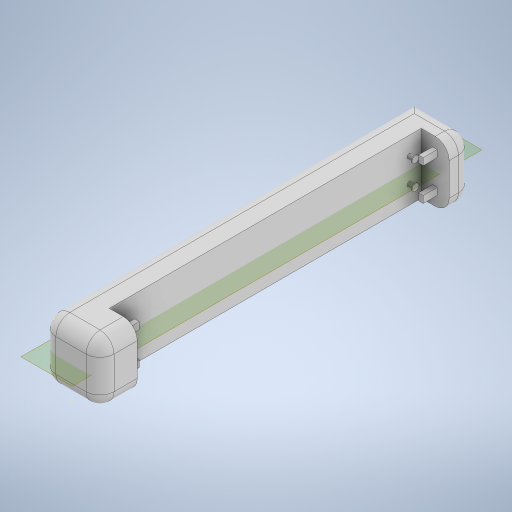
# Autodesk Inventor part: plane body
Saved by Autodesk Inventor 2023 (Build 270158000, 158)
## iProperties
Created: 2023-05-17
Part Number: plane body
Material: Generic
Document SubType Name: Modeling
Designer: Sujeet Kumar
Density: 1 g/cm^3
Appearance: Default
Author: Sujeet Kumar
Autodesk Inventor part; units mm, degrees
ref_plane "YZ Plane" through (0, 0, 0) normal (1, 0, 0) x (0, 1, 0)
sketch "Sketch1" plane through (0, 0, 0) normal (1, 0, 0) x (0, 1, 0)
  line L0 (0, 0) -> (130, 0)
  line L1 (130, 0) -> (130, -800)
  line L2 (130, -800) -> (0, -800)
  line L3 (0, -800) -> (0, 0)
  dimension "d0" = 130
  dimension "d1" = 800
  constraints: 8 end point, 2 parallel, 1 horizontal, 1 perpendicular
  measures "d0" distance of L1.end L2.end
  measures "d1" distance of L0.end L1.end
extrude "Extrusion1" add sketch "Sketch1" along normal blind 100 and the other way blind 25
sketch "Sketch2" plane through (-25, 130, 0) normal (0, 1, 0) x (1, 0, 0)
  line L0 (125, 800) -> (125, 0) projected
  line L1 (125, 80) -> (65, 80)
  line L2 (65, 80) -> (65, 750)
  line L3 (65, 750) -> (125, 750)
  line L4 (125, 750) -> (125, 80)
  line L5 (25, 0) -> (125, 0) projected
  line L6 (0, 800) -> (125, 800) projected
  point P0 (95, 80)
  point P1 (125, 750)
  dimension "d4" = 60
  dimension "d5" = 80
  dimension "d6" = 50
  constraints: 8 end point, 2 parallel, 1 horizontal, 1 midpoint, 1 perpendicular, 1 point on line
  measures "d4" distance of L2.end L3.end
  measures "d5" distance from line of point (95, 80) L5
  measures "d6" distance between parallel lines of L6 L3
extrude "Extrusion2" cut sketch "Sketch2" against normal blind 1000
sketch "Sketch3" plane through (100, 130, -80) normal (0, 0, -1) x (-1, 0, 0)
  line L0 (60, 0) -> (60, -130) projected
  line L1 (35.7484, -107.699) -> (25.7484, -107.699)
  line L2 (25.7484, -107.699) -> (25.7484, -92.699)
  line L3 (25.7484, -92.699) -> (35.7484, -92.699)
  line L4 (35.7484, -92.699) -> (35.7484, -107.699)
  point P0 (100, -130)
  dimension "d10" = 10
  dimension "d11" = 15
  constraints: 8 end point, 2 parallel, 1 horizontal, 1 perpendicular
  measures "d10" distance of L2.end L3.end
  measures "d11" distance of L1.end L2.end
extrude "Extrusion3" add sketch "Sketch3" along normal blind 30
sketch "Sketch4" plane through (-25, 0, -800) normal (0, -1, 0) x (1, 0, 0)
  line L0 (89.2516, 720) -> (89.2516, 690) projected
  line L1 (89.2516, 690) -> (74.8758, 690)
  line L2 (60.5, 690) -> (89.2516, 690) projected
  line L3 (74.8758, 690) -> (89.2516, 659.171)
  line L4 (74.8758, 690) -> (108.8918, 690) construction
  point P0 (25, 800)
  point P1 (50.5, 720)
  dimension "d14" = 115
  constraints: 6 end point, 1 equal length, 1 horizontal, 1 midpoint, 2 other
  measures "d14" angle of L4 L3
extrude "Extrusion4" [suppressed]
ref_plane "Work Plane1" through (-25, 65, -800) normal (0, -1, 0) x (1, 0, 0)
mirror "Mirror1" about plane through (-25, 65, -800) normal (0, -1, 0) of "Extrusion3"
ref_plane "Work Plane3" through (70, 0, -415) normal (0, 0, 1) x (1, 0, 0)
ref_plane "Work Plane2" through (70, 0, -750) normal (0, 0, 1) x (1, 0, 0)
mirror "Mirror2" about plane through (70, 0, -415) normal (0, 0, 1) of "Extrusion3", "Mirror1"
sketch "Sketch5" plane through (40, 130, -80) normal (1, 0, 0) x (0, 0, -1)
  point P0 (-80, -130)
sketch "Sketch6" plane through (-25, 130, 0) normal (0, 1, 0) x (1, 0, 0)
  point P0 (25, 0)
sketch "Sketch7" plane through (40, 130, -80) normal (1, 0, 0) x (0, 0, -1)
  line L0 (0, 0) -> (670, 0) projected
  line L1 (0, 0) -> (25, 0)
  line L2 (25, 0) -> (25, -39)
  line L3 (25, -39) -> (0, -39)
  line L4 (0, -39) -> (0, 0)
  circle A0 centre (25, -39) radius 5
  point P0 (-80, -130)
  dimension "d19" = 25
  dimension "d20" = 39
  dimension "d21" = 10
  constraints: 8 end point, 2 parallel, 1 centre point, 1 coincident, 1 horizontal, 1 perpendicular
  measures "d19" distance of L2.end L3.end
  measures "d20" distance of L1.end L2.end
  measures "d21" diameter of A0
extrude "Extrusion5" add sketch "Sketch7" along normal blind 10.5 contours A0 L3 L2 | L2 L3 A0
sketch "Sketch8" plane through (50.5, 91, -105) normal (1, 0, 0) x (0, 0, -1)
  circle A0 centre (0, 0) radius 5 projected
  circle A1 centre (0, 0) radius 7.5
  point P0 (-105, -91)
  dimension "d24" = 15
  constraints: 1 centre point, 1 coincident
  measures "d24" diameter of A1
extrude "Extrusion6" add sketch "Sketch8" along normal blind 2 contours A0 | A1
mirror "Mirror3" about plane through (-25, 65, -800) normal (0, -1, 0) of "Extrusion6", "Extrusion5"
ref_plane "Work Plane5" through (40, 130, -415) normal (0, 0, 1) x (1, 0, 0)
mirror "Mirror4" about plane through (40, 130, -415) normal (0, 0, 1) of "Extrusion6", "Extrusion5", "Mirror3"
sketch "Sketch9" plane through (-25, 0, 0) normal (-1, 0, 0) x (0, 0, 1)
  line L0 (-800, 130) -> (-750, 130) projected
  line L1 (-800, 130) -> (-800, 69)
  line L2 (-800, 130) -> (-800, 0) projected
  line L3 (-800, 69) -> (-750, 69)
  line L4 (-750, 69) -> (-750, 61)
  line L5 (-750, 61) -> (-800, 61)
  line L6 (-800, 61) -> (-800, 69)
  point P0 (0, 0)
  dimension "d28" = 61
  dimension "d29" = 50
  dimension "d30" = 8
  constraints: 10 end point, 2 parallel, 1 horizontal, 1 perpendicular, 1 point on line
  measures "d28" distance of L0.start L1.end
  measures "d29" distance of L4.end L5.end
  measures "d30" distance of L3.end L4.end
extrude "Extrusion7" cut sketch "Sketch9" against normal blind 50
sketch "Sketch11" plane through (-25, 69, -800) normal (0, -1, 0) x (1, 0, 0)
  line L0 (-0.1116, -0.1925) -> (24.8884, -0.1925)
  line L1 (24.8884, -0.1925) -> (24.8884, 24.8075)
  line L2 (24.8884, 24.8075) -> (-0.1116, 24.8075)
  line L3 (-0.1116, 24.8075) -> (-0.1116, -0.1925)
  circle A0 centre (24.8884, 24.8075) radius 5
  point P0 (25, 800)
  dimension "d33" = 25
  dimension "d34" = 25
  dimension "d35" = 10
  constraints: 8 end point, 2 parallel, 1 centre point, 1 coincident, 1 horizontal, 1 perpendicular
  measures "d33" distance of L2.end L1.end
  measures "d34" distance of L1.end L0.end
  measures "d35" diameter of A0
extrude "Extrusion8" add sketch "Sketch11" along normal blind 8 contours A0 L2 L1 | L1 L2 A0
sketch "Sketch12" plane through (-25, 0, 0) normal (-1, 0, 0) x (0, 0, 1)
  line L0 (-750, 69) -> (-750, 61) projected
  line L1 (-750, 65) -> (-750, 70)
  line L2 (-750, 130) -> (-750, 0) projected
  line L3 (-750, 70) -> (-490, 70)
  line L4 (-490, 70) -> (-490, 60)
  line L5 (-490, 60) -> (-750, 60)
  line L6 (-750, 60) -> (-750, 70)
  point P0 (0, 0)
  dimension "d40" = 5
  dimension "d41" = 260
  dimension "d42" = 10
  constraints: 10 end point, 2 parallel, 1 horizontal, 1 midpoint, 1 perpendicular, 1 point on line
  measures "d40" distance of L1.start L1.end
  measures "d41" distance of L4.end L5.end
  measures "d42" distance of L3.end L4.end
extrude "Extrusion9" cut sketch "Sketch12" against normal blind 55
fillet "Fillet1" radius 30 13 edges at (-25, 65, 0) (37.5, 130, 0) (100, 65, 0) (37.5, 0, 0) (-25, 130, -400) (-25, 0, -400) (37.5, 130, -800) (37.5, 0, -800) (100, 65, -800) (100, 0, -775) (100, 130, -775) (100, 0, -40) (100, 130, -40)
ref_plane "Work Plane4" through (-25, 65, -800) normal (0, -1, 0) x (1, 0, 0)
ref_plane "Work Plane6" through (-25, 65, -30) normal (0, 1, 0) x (1, 0, 0)
ref_plane "Work Plane7" through (-25, 65, -30) normal (0, 1, 0) x (1, 0, 0)
body "Solid1"
